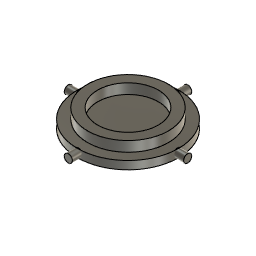
base v1 (Autodesk Fusion 360 design; units mm, degrees)
Autodesk Fusion 360 part; units mm, degrees
cylinder "CylinderPrimitive1" add diameter 100 height 8 placed x (1, 0, 0) y (0, 1, 0) z (0, 0, 1) at (0, 0, 0) makes body 1
cylinder "CylinderPrimitive2" add diameter 80 height 10 placed x (1, 0, 0) y (0, 1, 0) z (0, 0, 1) at (0, 0, 8) bodies 1
hole "Hole1" at (0, 0, 18) direction (0, 0, -1) diameter 60 depth 10 tip angle 180 bodies 1
cylinder "CylinderPrimitive3" add diameter 8 height 17 placed x (0, 1, 0) y (1, 0, 0) z (0, 0, -1) at (0, 0, 0) bodies 1
cylinder "CylinderPrimitive4" add diameter 8 height 10 placed x (0, 0, -1) y (0, 1, 0) z (1, 0, 0) at (0, 61, 25) separate body makes body 2
move_body "Move1" bodies 2 to x (1, 0, 0) y (0, 1, 0) z (0, 0, 1) at (50, -61, -21)
copy_body "CopyPasteBodies1" bodies 2 makes body 3
move_body "Move2" bodies 3 to x (1, 0, 0) y (0, 1, 0) z (0, 0, 1) at (-109, 0, 0)
move_body "Move3" bodies 2 to x (1, 0, 0) y (0, 1, 0) z (0, 0, 1) at (-1, 0, 0)
copy_body "CopyPasteBodies2" bodies 2 makes body 4
move_body "Move4" bodies 4 to x (0, 1, 0) y (-1, 0, 0) z (0, 0, 1) at (0, 0, 0)
copy_body "CopyPasteBodies3" bodies 3 makes body 5
move_body "Move5" bodies 5 to x (0, 1, 0) y (-1, 0, 0) z (0, 0, 1) at (0, 0, 0)
